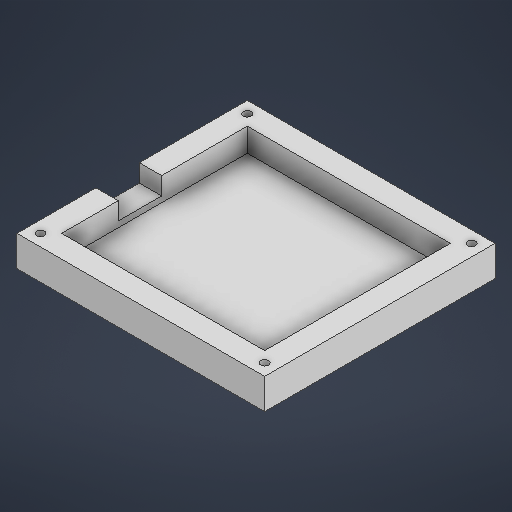
# Autodesk Inventor part: Bottom_Plate
Saved by Autodesk Inventor 2026 (Build 300175050, 175E)
## iProperties
Created: 2025-06-12
Part Number: Bottom_Plate
Material: Generic
Document SubType Name: Modeling
Designer: SaiAn
Density: 1 g/cm^3
Appearance: Default
Author: SaiAn
Autodesk Inventor part; units mm, degrees
ref_plane "YZ Plane" through (0, 0, 0) normal (1, 0, 0) x (0, 1, 0)
ref_plane "XZ Plane" through (0, 0, 0) normal (0, 1, 0) x (-1, 0, 0)
ref_plane "XY Plane" through (0, 0, 0) normal (0, 0, 1) x (1, 0, 0)
sketch "Sketch3" plane through (0, 0, 0) normal (0, 1, 0) x (-1, 0, 0)
  line L0 (0, 0) -> (86.5, 0)
  line L1 (86.5, 0) -> (86.5, -79.12)
  line L2 (86.5, -79.12) -> (0, -79.12)
  line L3 (0, -79.12) -> (0, 0)
  line L4 (-9.5, 9.5) -> (96, 9.5)
  line L5 (96, 9.5) -> (96, -88.62)
  line L6 (96, -88.62) -> (-9.5, -88.62)
  line L7 (-9.5, -88.62) -> (-9.5, 9.5)
  circle A0 centre (-4.5, 4.5) radius 1.7
  circle A1 centre (91, 4.5) radius 1.7
  circle A2 centre (-4.5, -83.62) radius 1.7
  circle A3 centre (91, -83.62) radius 1.7
  circle A4 centre (91, 4.5) radius 3
  circle A5 centre (-4.5, 4.5) radius 3
  circle A6 centre (-4.5, -83.62) radius 3
  circle A7 centre (91, -83.62) radius 3
  dimension "d0" = 86.5
  dimension "d1" = 79.12
  dimension "d2" = 105.5
  dimension "d3" = 98.12
  dimension "d4" = 9.5
  dimension "d5" = 9.5
  dimension "d6" = 3.4
  dimension "d7" = 3.4
  dimension "d8" = 3.4
  dimension "d9" = 3.4
  dimension "d10" = 5
  dimension "d11" = 5
  dimension "d12" = 5
  dimension "d13" = 5
  dimension "d14" = 5
  dimension "d15" = 5
  dimension "d16" = 5
  dimension "d17" = 5
  dimension "d18" = 6
  dimension "d19" = 6
  dimension "d20" = 6
  dimension "d21" = 6
  constraints: 16 end point, 8 centre point, 4 coincident, 4 parallel, 2 horizontal, 2 perpendicular
  measures "d0" distance of L1.end L2.end
  measures "d1" distance of L0.end L1.end
  measures "d2" distance of L5.end L6.end
  measures "d3" distance of L4.end L5.end
  measures "d4" distance between parallel lines of L1 L5
  measures "d5" distance between parallel lines of L6 L2
  measures "d6" diameter of A0
  measures "d7" diameter of A1
  measures "d8" diameter of A2
  measures "d9" diameter of A3
  measures "d10" distance from line of L5 A1.centre
  measures "d11" distance from line of L4 A1.centre
  measures "d12" distance from line of L4 A0.centre
  measures "d13" distance from line of L7 A0.centre
  measures "d14" distance from line of L7 A2.centre
  measures "d15" distance from line of L6 A2.centre
  measures "d16" distance from line of L5 A3.centre
  measures "d17" distance from line of L6 A3.centre
  measures "d18" diameter of A4
  measures "d19" diameter of A5
  measures "d20" diameter of A6
  measures "d21" diameter of A7
extrude "Extrusion1" add sketch "Sketch3" along normal blind 13 contours A4 | A5 | A6 | A7
sketch "Sketch4" plane through (-91, 13, 4.5) normal (0, 1, 0) x (1, 0, 0)
  point P0 (91, 4.5)
extrude "Extrusion2" cut sketch "Sketch3" along normal blind 3.1 contours A4 | A5 | A6 | A7
extrude "Extrusion3" add sketch "Sketch3" along normal blind 13 contours L4 L5 L6 L7
extrude "Extrusion4" add sketch "Sketch3" along normal blind 3 contours L0 L1 L2 L3
sketch "Sketch6" plane through (0, 13, 0) normal (0, 1, 0) x (1, 0, 0)
  line L0 (-96, 88.62) -> (-96, -9.5) projected
  line L1 (-96, 24.122) -> (-86.5, 24.122)
  line L2 (-86.5, 24.122) -> (-86.5, 42.622)
  line L3 (-86.5, 42.622) -> (-96, 42.622)
  line L4 (-96, 42.622) -> (-96, 24.122)
  point P0 (0, 0)
  dimension "d31" = 9.5
  dimension "d32" = 18.5
  constraints: 8 end point, 2 parallel, 1 horizontal, 1 perpendicular, 1 point on line
  measures "d31" distance of L3.end L2.end
  measures "d32" distance of L2.end L1.end
extrude "Extrusion5" cut sketch "Sketch6" against normal blind 7.5
body "Solid1"
